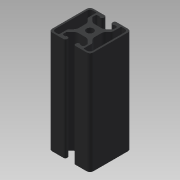
# Autodesk Inventor part: 40-4004-BLACK-FB
Saved by Autodesk Inventor 2013 (Build 170138000, 138)
## iProperties
Company: 80/20 Inc.
Created: 2014-04-23
Part Number: 40-4004-BLACK-FB
Material: Generic
Document SubType Name: Modeling
Designer: Ross Bowman
Density: 1 g/cm^3
Engineer: Ross Bowman
Catalog Web Link: 8020.net
Vendor: 80/20 Inc.
Material: 6105-T5 Aluminum
Author: Ross Bowman
Keywords: 80/20 , 8020 , T-Slot , Extrusion
Autodesk Inventor part; units mm, degrees
ref_plane "YZ Plane" through (0, 0, 0) normal (1, 0, 0) x (0, 1, 0)
ref_plane "XZ Plane" through (0, 0, 0) normal (0, 1, 0) x (-1, 0, 0)
ref_plane "XY Plane" through (0, 0, 0) normal (0, 0, 1) x (1, 0, 0)
sketch "Sketch1" plane through (0, 0, 0) normal (0, 0, 1) x (1, 0, 0)
  line L0 (9.015, -16.7025) -> (6.8938, -16.7025)
  line L1 (6.8938, -16.7025) -> (6.8938, -15.94)
  arc A0 (9.015, -16.7025) -> (10.285, -15.4325) centre (9.015, -15.4325) ccw
  line L2 (6.8938, -15.94) -> (5.6348, -15.94)
  line L3 (10.285, -12.9481) -> (10.285, -15.4325)
  arc A1 (5.6348, -15.94) -> (4.06, -17.5148) centre (5.6348, -17.5148) ccw
  arc A2 (10.285, -12.9481) -> (10.024, -12.3188) centre (9.396, -12.9481) ccw
  line L4 (4.06, -17.5148) -> (4.06, -18.4252)
  line L5 (6.7733, -9.0747) -> (10.024, -12.3188)
  arc A3 (4.06, -18.4252) -> (5.6348, -20) centre (5.6348, -18.4252) ccw
  arc A4 (6.7733, -9.0747) -> (3.4312, -7.7) centre (3.4312, -12.4498) ccw
  line L6 (5.6348, -20) -> (16.825, -20)
  line L7 (-3.4312, -7.7) -> (3.4312, -7.7)
  arc A5 (16.825, -20) -> (20, -16.825) centre (16.825, -16.825) ccw
  arc A6 (-3.4312, -7.7) -> (-6.7733, -9.0747) centre (-3.4312, -12.4498) ccw
  line L8 (20, -16.825) -> (20, 16.825)
  line L9 (-10.024, -12.3188) -> (-6.7733, -9.0747)
  arc A7 (20, 16.825) -> (16.825, 20) centre (16.825, 16.825) ccw
  arc A8 (-10.024, -12.3188) -> (-10.285, -12.9481) centre (-9.396, -12.9481) ccw
  line L10 (16.825, 20) -> (5.6348, 20)
  line L11 (-10.285, -15.4325) -> (-10.285, -12.9481)
  arc A9 (5.6348, 20) -> (4.06, 18.4252) centre (5.6348, 18.4252) ccw
  arc A10 (-10.285, -15.4325) -> (-9.015, -16.7025) centre (-9.015, -15.4325) ccw
  line L12 (4.06, 18.4252) -> (4.06, 17.5148)
  line L13 (-6.8938, -16.7025) -> (-9.015, -16.7025)
  arc A11 (4.06, 17.5148) -> (5.6348, 15.94) centre (5.6348, 17.5148) ccw
  line L14 (-6.8938, -15.94) -> (-6.8938, -16.7025)
  line L15 (5.6348, 15.94) -> (6.7718, 15.94)
  line L16 (-5.6348, -15.94) -> (-6.8938, -15.94)
  line L17 (6.7718, 15.94) -> (6.7718, 16.5629)
  arc A12 (-4.06, -17.5148) -> (-5.6348, -15.94) centre (-5.6348, -17.5148) ccw
  line L18 (6.7718, 16.5629) -> (9.015, 16.5629)
  line L19 (-4.06, -18.4252) -> (-4.06, -17.5148)
  arc A13 (10.285, 15.2929) -> (9.015, 16.5629) centre (9.015, 15.2929) ccw
  arc A14 (-5.6348, -20) -> (-4.06, -18.4252) centre (-5.6348, -18.4252) ccw
  line L20 (10.285, 15.2929) -> (10.285, 12.9795)
  line L21 (-16.825, -20) -> (-5.6348, -20)
  arc A15 (10.0407, 12.3673) -> (10.285, 12.9795) centre (9.396, 12.9795) ccw
  arc A16 (-20, -16.825) -> (-16.825, -20) centre (-16.825, -16.825) ccw
  line L22 (10.0407, 12.3673) -> (6.7505, 9.0839)
  line L23 (-20, 16.825) -> (-20, -16.825)
  arc A17 (3.4141, 7.7) -> (6.7505, 9.0839) centre (3.3992, 12.4498) ccw
  arc A18 (-16.825, 20) -> (-20, 16.825) centre (-16.825, 16.825) ccw
  line L24 (3.4141, 7.7) -> (-3.4141, 7.7)
  line L25 (-5.6348, 20) -> (-16.825, 20)
  arc A19 (-6.7505, 9.0839) -> (-3.4141, 7.7) centre (-3.3992, 12.4498) ccw
  arc A20 (-4.06, 18.4252) -> (-5.6348, 20) centre (-5.6348, 18.4252) ccw
  line L26 (-6.7505, 9.0839) -> (-10.0407, 12.3673)
  line L27 (-4.06, 17.5148) -> (-4.06, 18.4252)
  arc A21 (-10.285, 12.9795) -> (-10.0407, 12.3673) centre (-9.396, 12.9795) ccw
  arc A22 (-5.6348, 15.94) -> (-4.06, 17.5148) centre (-5.6348, 17.5148) ccw
  line L28 (-10.285, 12.9795) -> (-10.285, 15.2929)
  line L29 (-6.7718, 15.94) -> (-5.6348, 15.94)
  arc A23 (-9.015, 16.5629) -> (-10.285, 15.2929) centre (-9.015, 15.2929) ccw
  line L30 (-6.7718, 16.5629) -> (-6.7718, 15.94)
  line L31 (-9.015, 16.5629) -> (-6.7718, 16.5629)
  arc A24 (11.935, -17.7218) -> (12.5645, -18.35) centre (12.57, -17.715) ccw
  line L32 (11.935, -17.7218) -> (11.935, -10.9555)
  line L33 (15.5575, -18.35) -> (12.5645, -18.35)
  arc A25 (11.935, -10.9555) -> (11.0739, -8.7045) centre (8.7609, -10.8795) ccw
  arc A26 (15.5575, -18.35) -> (18.35, -15.5575) centre (15.556, -15.556) ccw
  line L34 (11.0739, -8.7045) -> (9.1386, -6.7731)
  line L35 (18.35, 15.5575) -> (18.35, -15.5575)
  arc A27 (7.685, -3.508) -> (9.1386, -6.7731) centre (12.4322, -3.3507) ccw
  arc A28 (18.35, 15.5575) -> (15.5575, 18.35) centre (15.556, 15.556) ccw
  line L36 (7.685, -3.508) -> (7.685, 3.2977)
  line L37 (12.566, 18.35) -> (15.5575, 18.35)
  arc A29 (9.033, 6.6995) -> (7.685, 3.2977) centre (12.434, 3.3839) ccw
  arc A30 (12.566, 18.35) -> (11.935, 17.7218) centre (12.57, 17.715) ccw
  line L38 (9.033, 6.6995) -> (10.9703, 8.6329)
  line L39 (11.935, 10.9555) -> (11.935, 17.7218)
  arc A31 (10.9703, 8.6329) -> (11.935, 10.9555) centre (8.7603, 10.9125) ccw
  circle A32 centre (0, 0) radius 3.4
  arc A33 (-11.0739, -8.7045) -> (-11.935, -10.9555) centre (-8.7609, -10.8795) ccw
  line L40 (-11.935, -10.9555) -> (-11.935, -17.7218)
  line L41 (-9.1386, -6.7731) -> (-11.0739, -8.7045)
  arc A34 (-12.5645, -18.35) -> (-11.935, -17.7218) centre (-12.57, -17.715) ccw
  arc A35 (-9.1386, -6.7731) -> (-7.685, -3.508) centre (-12.4322, -3.3507) ccw
  line L42 (-12.5645, -18.35) -> (-15.5575, -18.35)
  line L43 (-7.685, 3.2977) -> (-7.685, -3.508)
  arc A36 (-18.35, -15.5575) -> (-15.5575, -18.35) centre (-15.556, -15.556) ccw
  arc A37 (-7.685, 3.2977) -> (-9.033, 6.6995) centre (-12.434, 3.3839) ccw
  line L44 (-18.35, -15.5575) -> (-18.35, 15.5575)
  line L45 (-10.9703, 8.6329) -> (-9.033, 6.6995)
  arc A38 (-15.5575, 18.35) -> (-18.35, 15.5575) centre (-15.556, 15.556) ccw
  arc A39 (-11.935, 10.9555) -> (-10.9703, 8.6329) centre (-8.7603, 10.9125) ccw
  line L46 (-15.5575, 18.35) -> (-12.566, 18.35)
  line L47 (-11.935, 17.7218) -> (-11.935, 10.9555)
  arc A40 (-11.935, 17.7218) -> (-12.566, 18.35) centre (-12.57, 17.715) ccw
  constraints: 96 end point, 80 point on circle, 41 centre point
extrude "Extrusion1" add sketch "Sketch1" against normal blind 100
body "Solid1"
